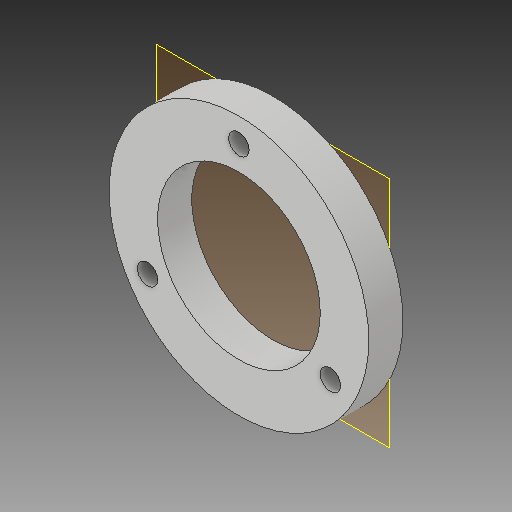
# Autodesk Inventor part: Проставка шестерни
Saved by Autodesk Inventor 2018.3 (Build 223284000, 284)
## iProperties
Created: 2018-07-22
Part Number: Проставка шестерни
Material: Типовые
Document SubType Name: Modeling
Designer: Leancher
Density: 1 g/cm^3
Appearance: По умолчанию
Author: Leancher
Autodesk Inventor part; units mm, degrees
ref_plane "YZ Plane" through (0, 0, 0) normal (1, 0, 0) x (0, 1, 0)
ref_plane "XZ Plane" through (0, 0, 0) normal (0, 1, 0) x (-1, 0, 0)
ref_plane "XY Plane" through (0, 0, 0) normal (0, 0, 1) x (1, 0, 0)
ref_plane "РабПлоскость1" through (0, 0, 0) normal (0, 0, 1) x (1, 0, 0)
sketch "Эскиз1" plane through (0, 0, 0) normal (0, 0, 1) x (1, 0, 0)
  circle A0 centre (0, 0) radius 11.9
  circle A1 centre (0, 0) radius 19
  circle A2 centre (-13.3801, -7.725) radius 1.5
  circle A3 centre (13.3801, -7.725) radius 1.5
  circle A4 centre (0, 15.45) radius 1.5
  dimension "d12" = 3
  dimension "d13" = 3
  dimension "d14" = 3
  constraints: 5 centre point, 1 coincident
  measures "d12" diameter of A2
  measures "d13" diameter of A3
  measures "d14" diameter of A4
extrude "Выдавливание1" add sketch "Эскиз1" along normal blind 5
